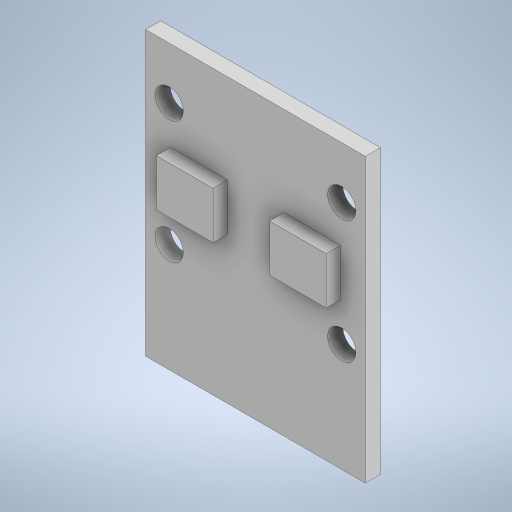
# Autodesk Inventor part: 모터 드라이버
Saved by Autodesk Inventor 2023.1 (Build 271208000, 208)
## iProperties
Created: 2022-09-03
Part Number: 모터 드라이버
Material: 일반
Document SubType Name: Modeling
Designer: fly01
Density: 1 g/cm^3
Appearance: 기본값
Author: fly01
Autodesk Inventor part; units mm, degrees
ref_plane "YZ Plane" through (0, 0, 0) normal (1, 0, 0) x (0, 1, 0)
ref_plane "XZ Plane" through (0, 0, 0) normal (0, 1, 0) x (-1, 0, 0)
ref_plane "XY Plane" through (0, 0, 0) normal (0, 0, 1) x (1, 0, 0)
sketch "스케치1" plane through (0, 0, 0) normal (0, 0, 1) x (1, 0, 0)
  line L0 (-11.65, 15) -> (11.65, 15)
  line L1 (11.65, 15) -> (11.65, -15)
  line L2 (11.65, -15) -> (-11.65, -15)
  line L3 (-11.65, -15) -> (-11.65, 15)
  line L4 (-11.65, 15) -> (11.65, -15) construction
  line L5 (11.65, 15) -> (-11.65, -15) construction
  line L6 (-9.15, 9.5) -> (9.15, 9.5) construction
  line L7 (9.15, 9.5) -> (9.15, -3.5) construction
  line L8 (9.15, -3.5) -> (-9.15, -3.5) construction
  line L9 (-9.15, -3.5) -> (-9.15, 9.5) construction
  line L10 (-9.15, 9.5) -> (9.15, -3.5) construction
  line L11 (9.15, 9.5) -> (-9.15, -3.5) construction
  line L12 (0, 3) -> (5.3972, 3)
  line L13 (0, 3) -> (0, 6.3473)
  circle A0 centre (-9.15, 9.5) radius 1.5
  circle A1 centre (-9.15, -3.5) radius 1.5
  circle A2 centre (9.15, 9.5) radius 1.5
  circle A3 centre (9.15, -3.5) radius 1.5
  point P0 (0, 0)
  dimension "d0" = 23.3
  dimension "d1" = 30
  dimension "d2" = 5.5
  dimension "d3" = 2.5
  dimension "d4" = 13
  dimension "d5" = 3
  constraints: 28 end point, 4 centre point, 4 midpoint, 4 parallel, 3 horizontal, 3 symmetric about line, 2 perpendicular, 1 coincident, 1 vertical, 1 vertical alignment, 3 other
  measures "d0" distance of L1.end L2.end
  measures "d1" distance of L0.end L1.end
  measures "d2" distance between parallel lines of L0 L6
  measures "d3" distance between parallel lines of L1 L7
  measures "d4" distance of L6.end L7.end
  measures "d5" diameter of A0
extrude "돌출1" add sketch "스케치1" along normal blind 1.6
sketch "스케치2" plane through (0, 0, 1.6) normal (0, 0, 1) x (1, 0, 0)
  line L0 (-9, 5.5) -> (-3, 5.5)
  line L1 (-3, 5.5) -> (-3, 0.5)
  line L2 (-3, 0.5) -> (-9, 0.5)
  line L3 (-9, 0.5) -> (-9, 5.5)
  line L4 (-9, 5.5) -> (-3, 0.5) construction
  line L5 (-3, 5.5) -> (-9, 0.5) construction
  line L6 (0, 0) -> (0, -2)
  line L7 (9, 5.5) -> (3, 5.5)
  line L8 (3, 5.5) -> (3, 0.5)
  line L9 (3, 0.5) -> (9, 0.5)
  line L10 (9, 0.5) -> (9, 5.5)
  line L11 (9, 5.5) -> (3, 0.5) construction
  line L12 (3, 5.5) -> (9, 0.5) construction
  point P0 (-6, 3)
  point P1 (6, 3)
  dimension "d8" = 6
  dimension "d9" = 5
  dimension "d10" = 6
  dimension "d11" = 3
  constraints: 26 end point, 5 symmetric about line, 2 midpoint, 2 parallel, 1 horizontal, 1 perpendicular, 1 vertical
  measures "d8" distance of L0.start L0.end
  measures "d9" distance of L2.end L0.start
  measures "d10" horizontal distance of L6.start point (-6, 3)
  measures "d11" vertical distance of L6.start point (-6, 3)
extrude "돌출2" add sketch "스케치2" along normal blind 1.5
